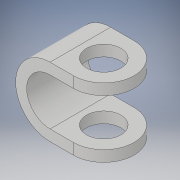
# Autodesk Inventor part: 410571040練習三
Saved by Autodesk Inventor 2017 (Build 210142000, 142)
## iProperties
Part Number: 410571040練習三
Material: 一般
Document SubType Name: Modeling
Designer: user
Density: 1 g/cm^3
Appearance: 預設
Author: user
Autodesk Inventor part; units mm, degrees
ref_plane "YZ Plane" through (0, 0, 0) normal (1, 0, 0) x (0, 1, 0)
ref_plane "XZ Plane" through (0, 0, 0) normal (0, 1, 0) x (-1, 0, 0)
ref_plane "XY Plane" through (0, 0, 0) normal (0, 0, 1) x (1, 0, 0)
sketch "草圖1" plane through (0, 0, 0) normal (0, 0, 1) x (1, 0, 0)
  arc A0 (0, 17) -> (0, -17) centre (0, 0) ccw
  arc A1 (0, 25) -> (0, -25) centre (0, 0) ccw
  line L0 (0, 27.0608) -> (0, -29.1984) construction
  line L1 (0, 25) -> (28, 25)
  line L2 (0, 17) -> (28, 17)
  line L3 (28, 25) -> (39, 25)
  line L4 (28, 17) -> (39, 17)
  line L5 (39, 17) -> (39, 25)
  line L6 (0, 0) -> (33.5, 0) construction
  line L7 (0, -25) -> (28, -25)
  line L8 (0, -17) -> (28, -17)
  line L9 (28, -25) -> (39, -25)
  line L10 (28, -17) -> (39, -17)
  line L11 (39, -17) -> (39, -25)
  dimension "d0" = 34
  dimension "d1" = 50
  dimension "d2" = 28
  dimension "d3" = 11
  dimension "d4" = 11
  dimension "d5" = 34
  constraints: 24 end point, 5 horizontal, 4 point on circle, 4 point on line, 4 symmetric about line, 2 centre point, 2 coincident, 1 perpendicular, 1 vertical
  measures "d0" diameter of A0
  measures "d1" diameter of A1
  measures "d2" distance of L1.start L1.end
  measures "d3" distance of L1.end L3.end
  measures "d4" distance of L2.end L4.end
  measures "d5" distance between parallel lines of L2 L8
extrude "擠出1" add sketch "草圖1" along normal mid plane 44
fillet "圓角1" radius 22 4 edges at (39, 21, 22) (39, 21, -22) (39, -21, 22) (39, -21, -22)
sketch "草圖2" plane through (0, 25, 22) normal (0, 1, 0) x (1, 0, 0)
  arc A0 (17, 0) -> (17, 44) centre (17, 22) ccw projected
  circle A1 centre (17, 22) radius 12.5
  point P0 (0, 22)
  dimension "d9" = 25
  constraints: 1 centre point, 1 coincident
  measures "d9" diameter of A1
extrude "擠出2" cut sketch "草圖2" against normal blind 60
